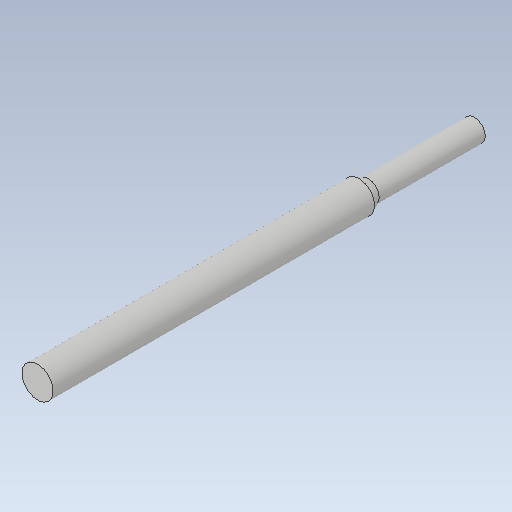
# Autodesk Inventor part: SMC_CJ1KB10-45(円柱)
Saved by Autodesk Inventor 2020 (Build 240168000, 168)
## iProperties
Created: 2018-04-28
Part Number: SMC_CJ1KB10-45(円柱)
Material: 一般
Document SubType Name: Modeling
Designer: Take
Density: 1 g/cm^3
Appearance: 既定
Author: Take
Autodesk Inventor part; units mm, degrees
ref_plane "YZ Plane" through (0, 0, 0) normal (1, 0, 0) x (0, 1, 0)
ref_plane "XZ Plane" through (0, 0, 0) normal (0, 1, 0) x (-1, 0, 0)
ref_plane "XY Plane" through (0, 0, 0) normal (0, 0, 1) x (1, 0, 0)
sketch "スケッチ1" plane through (0, 0, 0) normal (0, 1, 0) x (-1, 0, 0)
  line L0 (0, 0) -> (2.5, 0)
  line L1 (2.5, 0) -> (2.5, -51.5)
  line L2 (1.75, -53) -> (2.5, -51.5)
  line L3 (1.75, -53) -> (1.75, -70)
  line L4 (1.75, -70) -> (0, -70)
  line L5 (0, -70) -> (0, 0)
  point P0 (1.75, -51.5)
  point P1 (1.75, -51.5)
  dimension "d0" = 2.5
  dimension "d1" = 51.5
  dimension "d2" = 0.75
  dimension "d3" = 1.5
  dimension "d4" = 17
  constraints: 12 end point, 3 perpendicular, 1 coincident, 1 horizontal, 1 vertical
  measures "d0" distance of L0.start L0.end
  measures "d1" distance of L0.end L1.end
  measures "d2" distance of L1.end point (1.75, -51.5)
  measures "d3" distance of L2.start point (1.75, -51.5)
  measures "d4" distance of L2.start L3.end
revolve "回転1" add sketch "スケッチ1" angle 360 about axis through (0, 0, -70) along (0, 0, 1)
